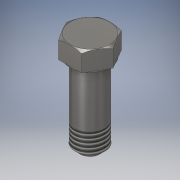
# Autodesk Inventor part: Hinge Pin
Saved by Autodesk Inventor 2018 (Build 220112000, 112)
## iProperties
Created: 2016-10-27
Part Number: Hinge Pin
Material: Steel, Carbon
Document SubType Name: Modeling
Designer: Joey
Density: 7.85 g/cm^3
Appearance: Semi-Polished
Mass: 8.75551 g
Surface Area: 8.6781 cm^2
Volume: 1.11535 cm^3
Author: Joey
Autodesk Inventor part; units mm, degrees
ref_plane "YZ Plane" through (0, 0, 0) normal (1, 0, 0) x (0, 1, 0)
ref_plane "XZ Plane" through (0, 0, 0) normal (0, 1, 0) x (-1, 0, 0)
ref_plane "XY Plane" through (0, 0, 0) normal (0, 0, 1) x (1, 0, 0)
sketch "Sketch1" plane through (0, 0, 0) normal (0, 0, 1) x (1, 0, 0)
  line L0 (0, 0) -> (9.525, 0)
  line L1 (9.525, 0) -> (9.525, -50.8)
  line L2 (9.525, -50.8) -> (0, -50.8)
  line L3 (0, -50.8) -> (0, 0)
  dimension "d0" = 19.05
  dimension "d1" = 50.8
  constraints: 8 end point, 2 parallel, 1 horizontal, 1 perpendicular
  measures "d0" diameter of L1 L3
  measures "d1" distance of L2.end L0.start
revolve "Revolution1" add sketch "Sketch1" angle 360 about axis through (0, -50.8, 0) along (0, 1, 0)
chamfer "Chamfer1" distance 3.175 angle 45 1 edges at (-9.525, -50.8, 0)
sketch "Sketch2" plane through (0, 0, 0) normal (0, 1, 0) x (1, 0, 0)
  circle A0 centre (0, 0) radius 12.7
  dimension "d6" = 25.4
  constraints: 1 centre point, 1 coincident
  measures "d6" diameter of A0
extrude "Extrusion1" add sketch "Sketch2" along normal blind 12.7
sketch "Sketch3" plane through (0, 12.7, 0) normal (0, 1, 0) x (1, 0, 0)
  line L0 (14.6647, 0) -> (7.3323, -12.7)
  line L1 (7.3323, -12.7) -> (-7.3323, -12.7)
  line L2 (-7.3323, -12.7) -> (-14.6647, 0)
  line L3 (-14.6647, 0) -> (-7.3323, 12.7)
  line L4 (-7.3323, 12.7) -> (7.3323, 12.7)
  line L5 (7.3323, 12.7) -> (14.6647, 0)
  circle A0 centre (0, 0) radius 12.7 construction
  point P0 (0, 0)
  point P1 (0, 0)
  constraints: 12 end point, 1 coincident, 1 horizontal, 1 tangent, 13 other
extrude "Extrusion2" add sketch "Sketch3" against normal blind 11.938
sketch "Sketch4" plane through (0, 0, 0) normal (0, 0, 1) x (1, 0, 0)
  line L0 (12.465, 12.7) -> (14.6647, 12.7)
  line L1 (14.6647, 12.7) -> (14.6647, 11.43)
  line L2 (14.6647, 11.43) -> (12.465, 12.7)
  line L3 (0, -0.2588) -> (0, 1.5529) projected
  line L4 (7.3323, 0) -> (14.6647, 0) construction
  line L5 (7.3323, 12.7) -> (14.6647, 12.7) construction
  line L6 (7.3323, 12.7) -> (7.3323, 0.762) construction
  line L7 (14.6647, 12.7) -> (14.6647, 0.762) construction
  line L8 (14.6647, 12.7) -> (7.3323, 12.7) projected
  line L9 (10.9985, 0.762) -> (14.6647, 0.762) projected
  line L10 (7.3323, 0.762) -> (10.9985, 0.762) projected
  point P0 (0, 0)
  point P1 (16.2522, 7.9375)
  dimension "d11" = 30
  dimension "d17" = 1.27
  constraints: 6 end point, 2 collinear, 1 horizontal, 1 perpendicular
  measures "d11" angle of L2 L0
  measures "d17" distance of L0.end L1.end
revolve "Revolution2" cut sketch "Sketch4" angle 360 about axis through (0, -10, 0) along (0, 1, 0)
thread "Thread2" size "3/4-10 UNC" class "2A" standard "ANSI Unified Screw Threads" length 12.7
equation "\"diameter\" = 1.8542"
equation "\"length\" = 19.05"
body "Solid1"
